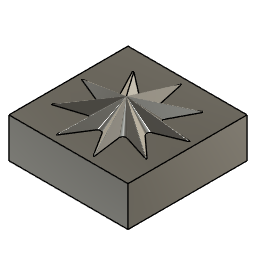
Star_CNC_milling v8 (Autodesk Fusion 360 design; units mm, degrees)
Autodesk Fusion 360 part; units mm, degrees
sketch "Sketch6" plane through (0, 0, 0) normal (0, 0, 1) x (1, 0, 0)
  circle A0 centre (0, 0) radius 50 construction
  circle A1 centre (0, 0) radius 20 construction
  line L0 (0, 0) -> (0, 50) construction
  line L1 (0, 0) -> (0, -20) construction
  line L2 (0, 0) -> (-32.1394, 38.3022) construction
  line L3 (0, 0) -> (12.8558, -15.3209) construction
  line L4 (0, 0) -> (-49.2404, 8.6824) construction
  line L5 (0, 0) -> (19.6962, -3.473) construction
  line L6 (0, 0) -> (-43.3013, -25) construction
  line L7 (0, 0) -> (17.3205, 10) construction
  line L8 (0, 0) -> (-17.101, -46.9846) construction
  line L9 (0, 0) -> (6.8404, 18.7939) construction
  line L10 (0, 0) -> (17.101, -46.9846) construction
  line L11 (0, 0) -> (-6.8404, 18.7939) construction
  line L12 (0, 0) -> (43.3013, -25) construction
  line L13 (0, 0) -> (-17.3205, 10) construction
  line L14 (0, 0) -> (49.2404, 8.6824) construction
  line L15 (0, 0) -> (-19.6962, -3.473) construction
  line L16 (0, 0) -> (32.1394, 38.3022) construction
  line L17 (0, 0) -> (-12.8558, -15.3209) construction
  line L18 (0.4884, 47.7719) -> (5.793, 23.5721)
  line L19 (-0.4884, 47.7719) -> (-5.793, 23.5721)
  arc A2 (0.4884, 47.7719) -> (-0.4884, 47.7719) centre (0, 47.6648) ccw
  line L20 (-31.0813, 36.2814) -> (-19.5895, 14.3336)
  line L21 (-30.333, 36.9093) -> (-10.7141, 21.7809)
  arc A3 (-30.333, 36.9093) -> (-31.0813, 36.2814) centre (-30.6384, 36.5134) ccw
  line L22 (-47.1309, 7.8145) -> (-24.2199, -1.6118)
  line L23 (-46.9613, 8.7765) -> (-22.208, 9.7983)
  arc A4 (-46.9613, 8.7765) -> (-47.1309, 7.8145) centre (-46.9407, 8.2769) ccw
  line L24 (-41.1275, -24.3089) -> (-17.5175, -16.8029)
  line L25 (-41.6159, -23.463) -> (-23.3105, -6.7691)
  arc A5 (-41.6159, -23.463) -> (-41.1275, -24.3089) centre (-41.279, -23.8324) ccw
  line L26 (-15.88, -45.0579) -> (-2.6185, -24.1318)
  line L27 (-16.7979, -44.7238) -> (-13.5058, -20.1692)
  arc A6 (-16.7979, -44.7238) -> (-15.88, -45.0579) centre (-16.3023, -44.7903) ccw
  line L28 (16.7979, -44.7238) -> (13.5058, -20.1692)
  line L29 (15.88, -45.0579) -> (2.6185, -24.1318)
  arc A7 (15.88, -45.0579) -> (16.7979, -44.7238) centre (16.3023, -44.7903) ccw
  line L30 (41.6159, -23.463) -> (23.3105, -6.7691)
  line L31 (41.1275, -24.3089) -> (17.5175, -16.8029)
  arc A8 (41.1275, -24.3089) -> (41.6159, -23.463) centre (41.279, -23.8324) ccw
  line L32 (46.9613, 8.7765) -> (22.208, 9.7983)
  line L33 (47.1309, 7.8145) -> (24.2199, -1.6118)
  arc A9 (47.1309, 7.8145) -> (46.9613, 8.7765) centre (46.9407, 8.2769) ccw
  line L34 (30.333, 36.9093) -> (10.7141, 21.7809)
  line L35 (31.0813, 36.2814) -> (19.5895, 14.3336)
  arc A10 (31.0813, 36.2814) -> (30.333, 36.9093) centre (30.6384, 36.5134) ccw
  arc A11 (5.793, 23.5721) -> (10.7141, 21.7809) centre (8.8211, 24.2358) ccw
  arc A12 (19.5895, 14.3336) -> (22.208, 9.7983) centre (22.3359, 12.8956) ccw
  arc A13 (24.2199, -1.6118) -> (23.3105, -6.7691) centre (25.3994, -4.4786) ccw
  arc A14 (17.5175, -16.8029) -> (13.5058, -20.1692) centre (16.5783, -19.7572) ccw
  arc A15 (2.6185, -24.1318) -> (-2.6185, -24.1318) centre (0, -25.7912) ccw
  arc A16 (-13.5058, -20.1692) -> (-17.5175, -16.8029) centre (-16.5783, -19.7572) ccw
  arc A17 (-23.3105, -6.7691) -> (-24.2199, -1.6118) centre (-25.3994, -4.4786) ccw
  arc A18 (-22.208, 9.7983) -> (-19.5895, 14.3336) centre (-22.3359, 12.8956) ccw
  arc A19 (-10.7141, 21.7809) -> (-5.793, 23.5721) centre (-8.8211, 24.2358) ccw
  dimension "d23" = 100
  dimension "d24" = 40
  dimension "d26" = 360
  dimension "d27" = 0.5
  dimension "d30" = 3.1
  constraint coincident A0.centre A1.centre
  constraint coincident A0 L0.end
  constraint vertical L0
  constraint coincident A1 L1.end
  constraint parallel L0 L1
  constraint coincident L0.end L19
  constraint coincident L0.end L18
  constraint tangent L19 A2
  constraint tangent L18 A2
  constraint coincident L9.end L18
  constraint tangent L18 A11
  constraint tangent L34 A11
  constraint tangent L35 A12
  constraint tangent L32 A12
  constraint equal A11 A12
  constraint tangent L33 A13
  constraint tangent L30 A13
  constraint equal A11 A13
  constraint tangent L31 A14
  constraint tangent L28 A14
  constraint equal A11 A14
  constraint tangent L29 A15
  constraint tangent L26 A15
  constraint equal A11 A15
  constraint tangent L27 A16
  constraint tangent L24 A16
  constraint equal A11 A16
  constraint tangent L25 A17
  constraint tangent L22 A17
  constraint equal A11 A17
  constraint tangent L23 A18
  constraint tangent L20 A18
  constraint equal A11 A18
  constraint coincident L11.end L19
  constraint tangent L21 A19
  constraint tangent L19 A19
  constraint equal A11 A19
  measures "d23" diameter of A0
  measures "d24" diameter of A1
  measures "d27" radius of A2
  measures "d30" radius of A11
ref_plane "Arbeitsebene2" through (0, 0, 15) normal (0, 0, 1) x (1, 0, 0)
sketch "Skizze4" plane through (0, 0, 15) normal (0, 0, 1) x (1, 0, 0)
loft "Loft2" add profiles "Sketch6" section 1 section 2 point at (0, 0, 15) makes body 1
box "BoxPrimitive3" add length 105 width 105 height 35 placed x (0, 1, 0) y (-1, 0, 0) z (0, 0, 1) at (228.724, -8.6065, 0) separate body makes body 2
move_body "Move3" bodies 1 to x (1, 0, 0) y (0, 1, 0) z (0, 0, 1) at (176.2213, 42.4787, 35)
combine "Combine2" operation add target body 2 tool bodies 1
